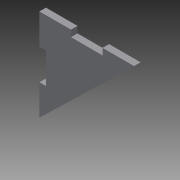
# Autodesk Inventor part: AngleSide
Saved by Autodesk Inventor 2013 (Build 170138000, 138)
## iProperties
Created: 2013-04-21
Part Number: AngleSide
Material: Generic
Document SubType Name: Modeling
Designer: fuji
Density: 1 g/cm^3
Author: fuji
Autodesk Inventor part; units mm, degrees
ref_plane "YZ Plane" through (0, 0, 0) normal (1, 0, 0) x (0, 1, 0)
ref_plane "XZ Plane" through (0, 0, 0) normal (0, 1, 0) x (-1, 0, 0)
ref_plane "XY Plane" through (0, 0, 0) normal (0, 0, 1) x (1, 0, 0)
sketch "Sketch1" plane through (0, 0, 0) normal (0, 0, 1) x (1, 0, 0)
  line L0 (0, 0) -> (45.72, 0)
  line L1 (45.72, 0) -> (45.72, 44.45)
  line L2 (45.72, 44.45) -> (0, 44.45)
  line L3 (0, 44.45) -> (0, 0)
  dimension "d0" = 45.72
  dimension "d1" = 44.45
  constraints: 8 end point, 2 parallel, 1 horizontal, 1 perpendicular
  measures "d0" distance of L2.end L1.end
  measures "d1" distance of L1.end L0.end
extrude "Extrusion1" add sketch "Sketch1" along normal blind 3.1496
sketch "Sketch2" plane through (0, 0, 3.1496) normal (0, 0, 1) x (1, 0, 0)
  line L0 (45.72, 44.45) -> (0, 44.45) projected
  line L1 (0, 44.45) -> (0, 0) projected
  line L2 (15.24, 44.45) -> (30.48, 44.45)
  line L3 (30.48, 44.45) -> (30.48, 41.3004)
  line L4 (30.48, 41.3004) -> (15.24, 41.3004)
  line L5 (15.24, 41.3004) -> (15.24, 44.45)
  line L6 (0, 29.6333) -> (3.1496, 29.6333)
  line L7 (3.1496, 29.6333) -> (3.1496, 14.8167)
  line L8 (3.1496, 14.8167) -> (0, 14.8167)
  line L9 (0, 14.8167) -> (0, 29.6333)
  dimension "d4" = 15.24
  dimension "d5" = 3.1496
  dimension "d6" = 15.24
  dimension "d7" = 3.1496
  dimension "d8" = 14.8167
  dimension "d9" = 14.8167
  constraints: 16 end point, 4 parallel, 2 horizontal, 2 perpendicular, 2 point on line
  measures "d4" distance of L3.end L4.end
  measures "d5" distance of L2.end L3.end
  measures "d6" distance between parallel lines of L5 L1
  measures "d7" distance of L7.end L8.end
  measures "d8" distance of L6.end L7.end
  measures "d9" distance between parallel lines of L6 L0
extrude "Extrusion2" cut sketch "Sketch2" against normal blind 3.1496
sketch "Sketch3" plane through (0, 0, 3.1496) normal (0, 0, 1) x (1, 0, 0)
  line L0 (0, 0) -> (45.72, 0) projected
  line L1 (45.72, 0) -> (45.72, 44.45) projected
  line L2 (45.72, 44.45) -> (0, 0)
  line L3 (45.72, 0) -> (45.72, 44.45)
  constraints: 4 end point, 1 collinear
extrude "Extrusion3" cut sketch "Sketch3" against normal blind 3.1496
equation "\"d0\" = angleLength"
equation "\"d1\" = angleHeight"
equation "\"d2\" = thick"
equation "\"d4\" = 0.333333 * angleLength"
equation "\"d5\" = thick"
equation "\"d6\" = 0.333333 * angleLength"
equation "\"d7\" = thick"
equation "\"d8\" = 0.333333 * angleHeight"
equation "\"d9\" = 0.333333 * angleHeight"
equation "\"d10\" = thick"
equation "\"d12\" = thick"
equation "\"thick\" = 3.1496"
equation "\"angleLength\" = 45.72"
equation "\"angleHeight\" = 44.45"
body "Solid1"
